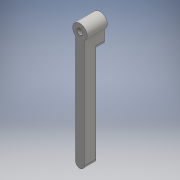
# Autodesk Inventor part: Traba
Saved by Autodesk Inventor 2016 (Build 200138000, 138)
## iProperties
Created: 2015-09-03
Part Number: Traba
Material: Generic
Document SubType Name: Modeling
Designer: amatiasq
Density: 1 g/cm^3
Appearance: Default
Mass: 0.61454 g
Surface Area: 7.48414 cm^2
Volume: 0.61454 cm^3
Author: amatiasq
Autodesk Inventor part; units mm, degrees
ref_plane "YZ Plane" through (0, 0, 0) normal (1, 0, 0) x (0, 1, 0)
ref_plane "XZ Plane" through (0, 0, 0) normal (0, 1, 0) x (-1, 0, 0)
ref_plane "XY Plane" through (0, 0, 0) normal (0, 0, 1) x (1, 0, 0)
sketch "Sketch1" plane through (0, 0, 0) normal (0, 1, 0) x (-1, 0, 0)
  line L0 (0, 0) -> (-3, 0)
  line L1 (-3, 0) -> (-3, -39)
  line L2 (-3, -39) -> (0, -39)
  line L3 (0, -39) -> (0, 0)
  circle A0 centre (-1.5, 2) radius 2.5
  circle A1 centre (-1.5, 2) radius 1
  dimension "d0" = 39
  dimension "d1" = 3
  dimension "d2" = 5
  dimension "d3" = 2
  constraints: 8 end point, 2 centre point, 2 parallel, 2 point on circle, 1 concentric, 1 horizontal, 1 perpendicular
  measures "d0" distance of L2.end L0.start
  measures "d1" distance of L0.start L0.end
  measures "d2" diameter of A0
  measures "d3" diameter of A1
extrude "Base" add sketch "Sketch1" along normal blind 4
sketch "Sketch2" plane through (0, 4, 0) normal (0, 1, 0) x (1, 0, 0)
  line L0 (0, 39) -> (0, 0) projected
  line L1 (3, 0) -> (3, 39) projected
  circle A0 centre (1.5, -2) radius 1 projected
  arc A1 (0, 0) -> (3, 0) centre (1.5, -2) ccw projected
  line L2 (3, 0) -> (3, 39) projected
  line L3 (3, 39) -> (0, 39) projected
  line L4 (0, 39) -> (0, 0) projected
  line L5 (0, 5) -> (3, 5)
  dimension "d8" = 5
  constraints: 2 end point, 2 point on line, 1 perpendicular
  measures "d8" distance from line of L5 L0.end
extrude "Superior" add sketch "Sketch2" along normal blind 3 contours L5 L1 A1 L0
fillet "Biselado" radius 1.5 4 edges at (3, 5.5, -5) (0, 5.5, -5) (3, 2, -39) (0, 2, -39)
equation "\"d0\" = traba_largo"
equation "\"d1\" = traba_ancho"
equation "\"d2\" = traba_diametro"
equation "\"d3\" = traba_diametro_perforacion"
equation "\"d4\" = traba_alto"
equation "\"d8\" = traba_top_largo"
equation "\"d9\" = traba_top_alto"
equation "\"d11\" = 0.5 * traba_ancho"
equation "\"base_alto\" = 3"
equation "\"deslizador_alto\" = 3"
equation "\"deslizador_alto_1\" = 3"
equation "\"deslizador_interruptor_ancho\" = 7"
equation "\"deslizador_interruptor_largo\" = 5"
equation "\"deslizador_largo\" = 144"
equation "\"deslizador_saliente\" = 5"
equation "\"deslizador_soporte_alto\" = 4"
equation "\"deslizador_soporte_ancho\" = 5"
equation "\"deslizador_tope_alto\" = 5"
equation "\"hoja_alto\" = 3"
equation "\"hoja_cola_biselado\" = 1"
equation "\"hoja_filo_biselado\" = 0.5"
equation "\"hoja_stop_biselado\" = 2"
equation "\"hoja_stop_largo\" = 5"
equation "\"hoja_stop_posicion\" = 5"
equation "\"hoja_stop_saliente\" = 5"
equation "\"margen\" = 0.3"
equation "\"muros_grosor\" = 3"
equation "\"rail_alto\" = 1.5"
equation "\"rail_grosor\" = 5"
equation "\"tirador_agarre_largo\" = 3"
equation "\"traba_largo\" = 39"
equation "\"traba_ancho\" = 3"
equation "\"traba_diametro\" = 5"
equation "\"traba_diametro_perforacion\" = 2"
equation "\"traba_alto\" = 4"
equation "\"traba_top_largo\" = 5"
equation "\"traba_top_alto\" = 3"
equation "\"base_separacion_agujeros\" = 4"
equation "\"base_agujeros_separacion\" = 3.5"
equation "\"base_agujeros_diametro\" = 2"
body "Solid1"
